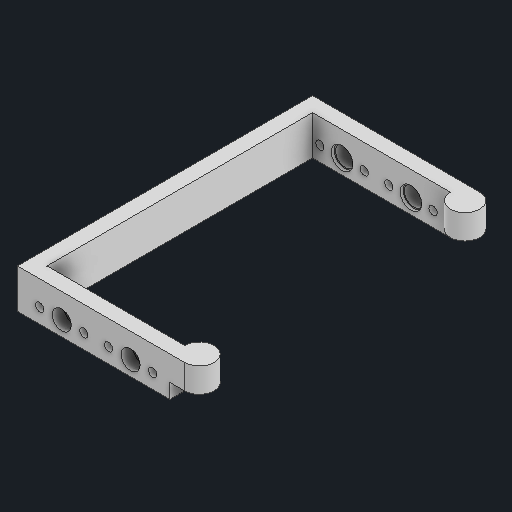
# Autodesk Inventor part: bmw
Saved by Autodesk Inventor 2026.2 (Build 302298010, 298A)
## iProperties
Created: 2026-04-27
Part Number: bmw
Material: Ogólny
Document SubType Name: Modeling
Designer: karol
Density: 1 g/cm^3
Appearance: Domyślna
Author: karol
Autodesk Inventor part; units mm, degrees
ref_plane "YZ Plane" through (0, 0, 0) normal (1, 0, 0) x (0, 1, 0)
ref_plane "XZ Plane" through (0, 0, 0) normal (0, 1, 0) x (-1, 0, 0)
ref_plane "XY Plane" through (0, 0, 0) normal (0, 0, 1) x (1, 0, 0)
sketch "Szkic1" plane through (0, 0, 0) normal (0, 1, 0) x (-1, 0, 0)
  line L0 (0, 0) -> (37, 0)
  line L1 (37, 0) -> (37, -3)
  line L2 (37, -3) -> (0, -3)
  line L3 (0, -3) -> (0, 0)
  line L4 (37, 0) -> (34, 0)
  line L5 (34, 0) -> (34, -60)
  line L6 (34, -60) -> (37, -60)
  line L7 (37, -60) -> (37, 0)
  line L8 (37, -60) -> (0, -60)
  line L9 (0, -60) -> (0, -57)
  line L10 (0, -57) -> (37, -57)
  line L11 (37, -57) -> (37, -60)
  point P0 (34, -3)
  point P1 (34, -57)
  dimension "d0" = 37
  dimension "d1" = 3
  dimension "d2" = 3
  dimension "d3" = 60
  dimension "d4" = 37
  dimension "d5" = 3
  constraints: 24 end point, 6 parallel, 3 horizontal, 3 perpendicular
  measures "d0" distance of L1.end L2.end
  measures "d1" distance of L0.end L1.end
  measures "d2" distance of L6.end L5.end
  measures "d3" distance of L5.end L4.end
  measures "d4" distance of L9.end L10.end
  measures "d5" distance of L8.end L9.end
extrude "Wyciągnięcie proste1" add sketch "Szkic1" along normal blind 8
sketch "Szkic2" plane through (-37, 0, 0) normal (0, 0, 1) x (1, 0, 0)
  circle A0 centre (9, 3) radius 1.95
  line L0 (0, 0) -> (37, 0) projected
  line L1 (0, 0) -> (0, 8) projected
  circle A1 centre (4.5, 3) radius 0.85
  circle A2 centre (13.5, 3) radius 0.85
  circle A3 centre (18.5, 3) radius 0.85
  circle A4 centre (27.5, 3) radius 0.85
  circle A5 centre (23, 3) radius 1.95
  dimension "d8" = 3.9
  dimension "d9" = 3
  dimension "d10" = 9
  dimension "d11" = 1.7
  dimension "d12" = 1.7
  dimension "d13" = 1.7
  dimension "d14" = 1.7
  dimension "d15" = 4.5
  dimension "d16" = 3
  dimension "d17" = 13.5
  dimension "d18" = 3
  dimension "d19" = 5
  dimension "d20" = 3
  dimension "d21" = 3.9
  dimension "d22" = 4.5
  dimension "d23" = 3
  dimension "d24" = 4.5
  dimension "d25" = 3
  constraints: 6 centre point
  measures "d8" diameter of A0
  measures "d9" distance from line of L0 A0.centre
  measures "d10" distance from line of L1 A0.centre
  measures "d11" diameter of A1
  measures "d12" diameter of A2
  measures "d13" diameter of A3
  measures "d14" diameter of A4
  measures "d15" distance from line of L1 A1.centre
  measures "d16" distance from line of L0 A1.centre
  measures "d17" distance from line of L1 A2.centre
  measures "d18" distance from line of L0 A2.centre
  measures "d19" distance of A2.centre A3.centre
  measures "d20" distance from line of L0 A3.centre
  measures "d21" diameter of A5
  measures "d22" distance of A3.centre A5.centre
  measures "d23" distance from line of L0 A5.centre
  measures "d24" distance of A5.centre A4.centre
  measures "d25" distance from line of L0 A4.centre
sketch "Szkic3" plane through (0, 0, -60) normal (0, 0, -1) x (-1, 0, 0)
  circle A0 centre (28, 3) radius 1.95 projected
  circle A1 centre (32.5, 3) radius 0.85 projected
  circle A2 centre (23.5, 3) radius 0.85 projected
  circle A3 centre (18.5, 3) radius 0.85 projected
  circle A4 centre (14, 3) radius 1.95 projected
  circle A5 centre (9.5, 3) radius 0.85 projected
  point P0 (0, 0)
extrude "Wyciągnięcie proste2" cut sketch "Szkic3" against normal blind 3
extrude "Wyciągnięcie proste3" cut sketch "Szkic2" against normal blind 3
sketch "Szkic4" plane through (0, 8, 0) normal (0, 1, 0) x (1, 0, 0)
  line L0 (0, 0) -> (0, 3) projected
  line L1 (0, 0) -> (-6, 0)
  line L2 (-6, 0) -> (-6, 6)
  line L3 (-6, 6) -> (0, 6)
  line L4 (0, 6) -> (0, 0)
  line L5 (0, 60) -> (-37, 60) projected
  line L6 (0, 60) -> (-6, 60)
  line L7 (-6, 60) -> (-6, 54)
  line L8 (-6, 54) -> (0, 54)
  line L9 (0, 54) -> (0, 60)
  dimension "d30" = 6
  dimension "d31" = 6
  dimension "d32" = 6
  dimension "d33" = 6
  constraints: 16 end point, 4 parallel, 2 horizontal, 2 perpendicular
  measures "d30" distance of L2.end L3.end
  measures "d31" distance of L1.end L2.end
  measures "d32" distance of L8.end L7.end
  measures "d33" distance of L7.end L6.end
extrude "Wyciągnięcie proste4" add sketch "Szkic4" against normal blind 8
sketch "Szkic5" plane through (0, 0, 0) normal (0, -1, 0) x (1, 0, 0)
  line L0 (-6, -6) -> (0, -6) projected
  line L1 (0, -6) -> (-6, -6)
  line L2 (-6, -6) -> (-6, 0)
  line L3 (-6, 0) -> (0, 0)
  line L4 (0, 0) -> (0, -6)
  line L5 (0, -54) -> (-6, -54) projected
  line L6 (0, -60) -> (-37, -60) projected
  line L7 (0, -54) -> (-6, -54)
  line L8 (-6, -54) -> (-6, -60)
  line L9 (-6, -60) -> (0, -60)
  line L10 (0, -60) -> (0, -54)
  constraints: 16 end point, 4 parallel, 2 horizontal, 2 perpendicular, 2 point on line
extrude "Wyciągnięcie proste5" cut sketch "Szkic5" against normal blind 3
sketch "Szkic6" plane through (0, 3, 0) normal (0, -1, 0) x (1, 0, 0)
  circle A0 centre (-3, -3) radius 2
  circle A1 centre (-3, -57) radius 2
  line L0 (0, 0) -> (0, -6) projected
  line L1 (-6, 0) -> (0, 0) projected
  line L2 (-6, -54) -> (0, -54) projected
  line L3 (0, -54) -> (0, -60) projected
  point P0 (-3, -54)
  dimension "d38" = 4
  dimension "d39" = 4
  dimension "d40" = 3
  dimension "d41" = 3
  dimension "d42" = 3
  dimension "d43" = 3
  constraints: 2 centre point, 1 midpoint
  measures "d38" diameter of A0
  measures "d39" diameter of A1
  measures "d40" distance from line of L0 A0.centre
  measures "d41" distance from line of L1 A0.centre
  measures "d42" distance of point (-3, -54) A1.centre
  measures "d43" distance from line of L3 A1.centre
extrude "Wyciągnięcie proste6" cut sketch "Szkic6" against normal blind 4
sketch "Szkic7" plane through (-34, 0, -3) normal (0, 0, -1) x (-1, 0, 0)
  circle A0 centre (-6, 3) radius 1.95 projected
  circle A1 centre (-6, 3) radius 2.2
  circle A2 centre (-20, 3) radius 1.95 projected
  circle A3 centre (-20, 3) radius 2.2
  point P0 (-34, 0)
  dimension "d46" = 4.4
  dimension "d47" = 4.4
  constraints: 2 centre point, 2 coincident
  measures "d46" diameter of A1
  measures "d47" diameter of A3
extrude "Wyciągnięcie proste7" cut sketch "Szkic7" against normal blind 0.6 contours A0 | A1 | A2 | A3
sketch "Szkic8" plane through (-34, 0, -57) normal (0, 0, 1) x (1, 0, 0)
  circle A0 centre (20, 3) radius 2.2 projected
  circle A1 centre (20, 3) radius 2.2
  circle A2 centre (6, 3) radius 2.2 projected
  circle A3 centre (6, 3) radius 2.2
  point P0 (34, 0)
  dimension "d50" = 4.4
  dimension "d51" = 4.4
  constraints: 2 centre point, 2 coincident
  measures "d50" diameter of A1
  measures "d51" diameter of A3
extrude "Wyciągnięcie proste8" cut sketch "Szkic8" against normal blind 0.6
fillet "Fillet1" radius 3 4 edges at (0, 5.5, 0) (0, 5.5, -6) (0, 5.5, -54) (0, 5.5, -60)
fillet "Zaokrąglenie2" radius 3 2 edges at (-6, 5.5, -54) (-6, 5.5, -6)
